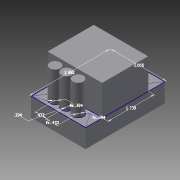
# Autodesk Inventor part: HobbyWing EZRUN 150A Pro 2
Saved by Autodesk Inventor 2015 SP1 (Build 190203100, 203)
## iProperties
Created: 2016-04-06
Part Number: HobbyWing EZRUN 150A Pro 2
Material: Generic
Document SubType Name: Modeling
Designer: doctor
Density: 1 g/cm^3
Appearance: Default
Author: doctor
Autodesk Inventor part; units mm, degrees
ref_plane "YZ Plane" through (0, 0, 0) normal (1, 0, 0) x (0, 1, 0)
ref_plane "XZ Plane" through (0, 0, 0) normal (0, 1, 0) x (-1, 0, 0)
ref_plane "XY Plane" through (0, 0, 0) normal (0, 0, 1) x (1, 0, 0)
sketch "Sketch2" plane through (0, 0, 0) normal (0, 1, 0) x (-1, 0, 0)
  line L0 (-26.1, 38) -> (26.1, 38)
  line L1 (26.1, 38) -> (26.1, -38)
  line L2 (26.1, -38) -> (-26.1, -38)
  line L3 (-26.1, -38) -> (-26.1, 38)
  line L4 (-26.1, 38) -> (26.1, -38) construction
  line L5 (26.1, 38) -> (-26.1, -38) construction
  line L6 (26.1, 22.085) -> (-26.1, 22.085)
  line L7 (-26.1, 22.085) -> (-26.1, -22.085)
  line L8 (-26.1, -22.085) -> (26.1, -22.085)
  line L9 (26.1, -22.085) -> (26.1, 22.085)
  line L10 (26.1, 22.085) -> (-26.1, -22.085) construction
  line L11 (-26.1, 22.085) -> (26.1, -22.085) construction
  line L12 (26.1, 38) -> (-26.1, 22.085) construction
  circle A0 centre (0, 30.0425) radius 5
  circle A1 centre (11, 30.0425) radius 5
  circle A2 centre (-11, 30.0425) radius 5
  point P0 (0, 0)
  dimension "d0" = 52.2
  dimension "d1" = 76
  dimension "d2" = 44.17
  dimension "OutCableDia" = 10
  dimension "d9" = 10
  dimension "d10" = 10
  dimension "d11" = 11
  dimension "d12" = 11
  constraints: 26 end point, 5 midpoint, 4 parallel, 3 centre point, 2 horizontal, 2 horizontal alignment, 2 perpendicular, 1 coincident, 1 point on line
  measures "d0" distance of L1.end L2.end
  measures "d1" distance of L0.end L1.end
  measures "d2" distance of L7.end L6.end
  measures "OutCableDia" diameter of A0
  measures "d9" diameter of A1
  measures "d10" diameter of A2
  measures "d11" distance of point (0, 30.043) A1.centre
  measures "d12" distance of point (0, 30.043) A2.centre
extrude "Extrusion1" add sketch "Sketch2" against normal blind 18 contours L0 L1 L6 L3 | L6 L1 L8 L3 | L8 L1 L2 L3 | A0 | A1 | A2
extrude "Extrusion2" add sketch "Sketch2" along normal blind 29 contours L6 L1 L8 L3
extrude "Extrusion3" add sketch "Sketch2" along normal blind 29 contours A0 | A1 | A2
equation "\"d9\" = OutCableDia"
equation "\"d10\" = OutCableDia"
equation "\"d12\" = d11"
body "Solid1"
